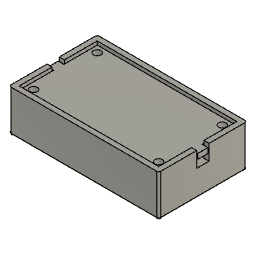
DC-DC Enclosure v1 (Autodesk Fusion 360 design; units mm, degrees)
Autodesk Fusion 360 part; units mm, degrees
sketch "Main geometry layout" plane through (0, 0, 0) normal (0, 0, 1) x (1, 0, 0)
  line L0 (0, 0) -> (61, 0) construction
  line L1 (61, 0) -> (61, 31) construction
  line L2 (61, 31) -> (0, 31) construction
  line L3 (0, 31) -> (0, 0) construction
  circle A0 centre (0, 0) radius 2.75
  circle A1 centre (61, 0) radius 2.75
  circle A2 centre (0, 31) radius 2.75
  circle A3 centre (61, 31) radius 2.75
  line L4 (64.5, 34.5) -> (-3.5, 34.5)
  line L5 (-3.5, 34.5) -> (-3.5, -3.5)
  line L6 (-3.5, -3.5) -> (64.5, -3.5)
  line L7 (64.5, -3.5) -> (64.5, 34.5)
  line L8 (0, 0) -> (9, 0) construction
  line L9 (9, 0) -> (9, 2) construction
  line L10 (9, 2) -> (0, 2) construction
  line L11 (0, 2) -> (0, 0) construction
  circle A4 centre (9, 2) radius 2
  circle A5 centre (29, 31) radius 1.5
  line L12 (-6, -6) -> (67, -6)
  line L13 (67, -6) -> (67, 37)
  line L14 (67, 37) -> (-6, 37)
  line L15 (-6, 37) -> (-6, -6)
  line L16 (-6, 18.5) -> (-3.5, 18.5)
  line L17 (-3.5, 18.5) -> (-3.5, 12.5)
  line L18 (-3.5, 12.5) -> (-6, 12.5)
  line L19 (-6, 12.5) -> (-6, 18.5)
  line L20 (30.5, -13.9919) -> (30.5, 45)
  line L21 (64.5, 18.5) -> (64.5, 12.5)
  line L22 (67, 18.5) -> (64.5, 18.5)
  line L23 (67, 12.5) -> (67, 18.5)
  line L24 (64.5, 12.5) -> (67, 12.5)
  line L25 (-3.5, 34.5) -> (-1.5, 34.5)
  line L26 (-1.5, 34.5) -> (-1.5, 22.5)
  line L27 (-1.5, 22.5) -> (-3.5, 22.5)
  line L28 (-3.5, 22.5) -> (-3.5, 34.5)
  line L29 (72.2627, 15.5) -> (-12, 15.5)
  line L30 (-3.5, -3.5) -> (-1.5, -3.5)
  line L31 (-1.5, -3.5) -> (-1.5, 8.5)
  line L32 (-1.5, 8.5) -> (-3.5, 8.5)
  line L33 (-3.5, 8.5) -> (-3.5, -3.5)
  line L34 (64.5, 34.5) -> (62.5, 34.5)
  line L35 (62.5, 22.5) -> (64.5, 22.5)
  line L36 (64.5, 22.5) -> (64.5, 34.5)
  line L37 (62.5, 34.5) -> (62.5, 22.5)
  line L38 (64.5, 8.5) -> (64.5, -3.5)
  line L39 (64.5, -3.5) -> (62.5, -3.5)
  line L40 (62.5, 8.5) -> (64.5, 8.5)
  line L41 (62.5, -3.5) -> (62.5, 8.5)
  circle A6 centre (9, 2) radius 4.5
  line L42 (18, -1.5) -> (40.5, -1.5)
  line L43 (40.5, -1.5) -> (40.5, 12.5)
  line L44 (40.5, 12.5) -> (18, 12.5)
  line L45 (18, 12.5) -> (18, -1.5)
  line L46 (-1.5, 22.5) -> (-1.5, 8.5)
  line L47 (62.5, 22.5) -> (62.5, 8.5)
  line L48 (13.5, 2) -> (13.5, -3.5)
  line L49 (4.5, 2) -> (4.5, -3.5)
  line L50 (2.75, 0) -> (2.75, -3.5)
  line L51 (2.75, 31) -> (2.75, 34.5)
  line L52 (58.25, 31) -> (58.25, 34.5)
  line L53 (58.25, 0) -> (58.25, -3.5)
  circle A7 centre (0, 0) radius 1.25
  circle A8 centre (61, 0) radius 1.25
  circle A9 centre (0, 31) radius 1.25
  circle A10 centre (61, 31) radius 1.25
  dimension "d1" = 61
  dimension "d2" = 31
  dimension "d6" = 5.5
  dimension "d9" = 61
  dimension "d10" = 31
  dimension "d11" = 3.5
  dimension "d16" = 9
  dimension "d17" = 2
  dimension "d18" = 4
  dimension "d19" = 3
  dimension "d20" = 29
  dimension "d21" = 6
  dimension "d22" = 6
  dimension "d31" = 2
  dimension "d32" = 12
  dimension "d35" = 2.5
  dimension "d40" = 22.5
  dimension "d41" = 14
  dimension "d42" = 18
  dimension "d43" = 2
  dimension "d50" = 2.5
  dimension "d53" = 61
  dimension "d54" = 31
  constraint horizontal L0
  constraint vertical L1
  constraint horizontal L2
  constraint vertical L3
  constraint coincident L0.start L3.end
  constraint horizontal L8
  constraint vertical L9
  constraint horizontal L10
  constraint vertical L11
  constraint coincident L9.end L10.start
  constraint coincident L2 A5.centre
  constraint horizontal L16
  constraint vertical L17
  constraint horizontal L18
  constraint vertical L19
  constraint coincident L15 L16.start
  constraint midpoint L15 L19
  constraint perpendicular L4 L20
  constraint symmetric L16.start L20 L22.start
  constraint symmetric L16.end L20 L21.start
  constraint symmetric L17.end L20 L21.end
  constraint symmetric L18.end L20 L23.start
  constraint horizontal L25
  constraint vertical L26
  constraint horizontal L27
  constraint vertical L28
  constraint perpendicular L21 L29
  constraint symmetric L4.end L29 L5.end
  constraint symmetric L25.end L29 L30.end
  constraint symmetric L26.end L29 L31.end
  constraint symmetric L27.end L29 L32.end
  constraint symmetric L4.end L20 L4.start
  constraint symmetric L20 L25.end L34.end
  constraint symmetric L20 L26.end L35.start
  constraint symmetric L20 L27.end L35.end
  constraint symmetric L20 L5.end L6.end
  constraint symmetric L20 L30.end L39.end
  constraint symmetric L20 L31.end L40.start
  constraint symmetric L20 L32.end L38.start
  constraint horizontal L42
  constraint vertical L43
  constraint horizontal L44
  constraint vertical L45
  constraint coincident A6 L48.start
  constraint coincident L6 L48.end
  constraint tangent A6 L48
  constraint perpendicular L6 L48
  constraint midpoint L10 L49.start
  constraint coincident L6 L49.end
  constraint tangent A6 L49
  constraint perpendicular L6 L49
  constraint coincident A0 L50.start
  constraint coincident L0 L50.start
  constraint coincident L6 L50.end
  constraint tangent A0 L50
  constraint symmetric L29 L50.start L51.start
  constraint symmetric L29 L50.end L51.end
  constraint symmetric L20 L50.start L53.start
  constraint symmetric L20 L50.end L53.end
  constraint symmetric L20 L51.start L52.start
  constraint symmetric L20 L51.end L52.end
  measures "d1" distance of L0.start L0.end
  measures "d2" distance of L0.start L2.end
  measures "d6" diameter of A0
  measures "d16" distance of L0.start L8.end
  measures "d17" distance of L0.start L10.end
  measures "d18" diameter of A4
  measures "d19" diameter of A5
  measures "d20" distance of L2.end A5.centre
  measures "d22" distance of L16.start L18.end
  measures "d31" distance of L4.end L25.end
  measures "d32" distance of L4.end L27.end
  measures "d40" distance of L42.start L42.end
  measures "d41" distance of L42.start L44.end
  measures "d42" distance of L0.start L45
  measures "d43" distance of L6 L42
  measures "d50" diameter of A7
extrude "Extrude1" add sketch "Main geometry layout" against normal blind 2.5 contours A0 L31 | A0 L6 L31 L50 | A0 L6 L20 L29 L31 A6 L42 L44 L45 L46 L48 L49 L50 | A0 L31 | A0 L5 L6 L30 L31 L32 L33 | L5 L6 L12 L15 L18 L20 L30 L33 | L5 L17 L29 L32 L46 | L6 A6 L48 L49 | A2 L4 L20 L26 L29 L46 L51 | L5 L17 L27 L29 L46 | A6 | L5 L15 L17 L18 L19 L29 | A1 L6 L20 L29 L41 L42 L43 L44 L47 L53 | A3 L4 L20 L29 L37 L47 L52 | L5 L15 L16 L17 L19 L29 | A2 L4 L5 L25 L26 L27 L28 | L6 L7 L12 L13 L20 L24 L38 L39 | L20 L42 L43 L44 | L20 L42 L44 L45 | L7 L21 L29 L35 L47 | L7 L21 L29 L40 L47 | L4 L5 L14 L15 L16 L20 L25 L28 | A2 L26 | A2 L26 | A1 L6 L41 L53 | L4 L7 L13 L14 L20 L22 L34 L36 | L7 L13 L21 L23 L24 L29 | L7 L13 L21 L22 L23 L29 | A3 L4 L7 L34 L35 L36 L37 | A1 L6 L7 L38 L39 L40 L41 | A2 L4 L26 L51 | A1 L41 | A3 L4 L37 L52 | A3 L37 | A3 L37 | A1 L41 | A7 | A8 | A9 | A10 makes body 1
extrude "Extrude2" add sketch "Main geometry layout" along normal blind 18 contours L5 L6 L12 L15 L18 L20 L30 L33 | L5 L15 L17 L18 L19 L29 | L5 L15 L16 L17 L19 L29 | L6 L7 L12 L13 L20 L24 L38 L39 | L4 L5 L14 L15 L16 L20 L25 L28 | L4 L7 L13 L14 L20 L22 L34 L36 | L7 L13 L21 L23 L24 L29 | L7 L13 L21 L22 L23 L29 bodies 1
sketch "Cable cutouts" plane through (0, 0, 18) normal (0, 0, 1) x (-1, 0, 0)
  line L0 (3.5, -34.5) -> (-64.5, -34.5)
  line L1 (-64.5, -34.5) -> (-64.5, 3.5)
  line L2 (-64.5, 3.5) -> (3.5, 3.5)
  line L3 (3.5, 3.5) -> (3.5, -34.5)
  line L4 (6, -37) -> (6, 6)
  line L5 (6, 6) -> (-67, 6)
  line L6 (-67, 6) -> (-67, -37)
  line L7 (-67, -37) -> (6, -37)
  line L8 (3.5, -12.5) -> (6, -12.5)
  line L9 (6, -12.5) -> (6, -18.5)
  line L10 (6, -18.5) -> (3.5, -18.5)
  line L11 (3.5, -18.5) -> (3.5, -12.5)
  line L12 (-64.5, -12.5) -> (-67, -12.5)
  line L13 (-67, -12.5) -> (-67, -18.5)
  line L14 (-64.5, -18.5) -> (-64.5, -12.5)
  line L15 (-67, -18.5) -> (-64.5, -18.5)
extrude "Extrude3" cut sketch "Cable cutouts" against normal blind 7.5 contours L3 L4 L8 L9 L10 L11 | L1 L6 L12 L13 L14 L15 bodies 1
fillet "Fillet1" radius 1 8 edges at (30.5, 37, -2.5) (-6, 37, 7.75) (67, 37, 7.75) (67, 15.5, -2.5) (67, -6, 7.75) (30.5, -6, -2.5) (-6, 15.5, -2.5) (-6, -6, 7.75) on bodies 1
extrude "Extrude4" add sketch "Main geometry layout" along normal blind 12 contours A0 L31 | A0 L6 L31 L50 | A0 L31 | A0 L5 L6 L30 L31 L32 L33 | A2 L4 L5 L25 L26 L27 L28 | A2 L26 | A2 L26 | A1 L6 L41 L53 | A3 L4 L7 L34 L35 L36 L37 | A1 L6 L7 L38 L39 L40 L41 | A2 L4 L26 L51 | A1 L41 | A3 L4 L37 L52 | A3 L37 | A3 L37 | A1 L41 | A7 | A8 | A9 | A10 bodies 1
extrude "Extrude5" add sketch "Main geometry layout" along normal blind 5 contours L6 A6 L48 L49 | A6 bodies 1
extrude "Extrude6" cut sketch "Main geometry layout" against normal blind 1.25 contours L20 L42 L43 L44 | L20 L42 L44 L45 bodies 1
fillet "Fillet2" radius 0.5 2 edges at (7.1353, 1.2768, -2.5) (27.6015, 30.4576, -2.5) on bodies 1
extrude "Extrude7" add sketch "Main geometry layout" along normal up to surface (10.5 mm away) contours L5 L17 L29 L32 L46 | L5 L17 L27 L29 L46 | L7 L21 L29 L35 L47 | L7 L21 L29 L40 L47 bodies 1
sketch "Mounting holes" plane through (0, 0, 12) normal (0, 0, 1) x (-1, 0, 0)
  arc A0 (1.5, -28.6951) -> (-2.75, -31) centre (0, -31) ccw
  line L0 (-2.75, -31) -> (-2.75, -34.5)
  line L1 (-2.75, -34.5) -> (3.5, -34.5)
  line L2 (3.5, -34.5) -> (3.5, -22.5)
  line L3 (3.5, -22.5) -> (1.5, -22.5)
  line L4 (1.5, -22.5) -> (1.5, -28.6951)
  circle A1 centre (0, -31) radius 1.25
  circle A2 centre (-61, -31) radius 1.25
  circle A3 centre (-61, 0) radius 1.25
  circle A4 centre (0, 0) radius 1.25
  point P0 (-61, 0)
extrude "Extrude8" cut sketch "Mounting holes" against normal blind 10 contours A1 | A2 | A3 | A4 bodies 1
sketch "Bottom lid" plane through (0, 0, 18) normal (0, 0, 1) x (-1, 0, 0)
  arc A0 (-66, 6) -> (-67, 5) centre (-66, 5) ccw
  line L0 (-67, 5) -> (-67, -12.5)
  line L1 (-67, -12.5) -> (-64.5, -12.5) construction
  line L2 (-64.5, -12.5) -> (-64.5, 3.5)
  line L3 (-64.5, 3.5) -> (3.5, 3.5) construction
  line L4 (3.5, 3.5) -> (3.5, -12.5)
  line L5 (3.5, -12.5) -> (6, -12.5)
  line L6 (6, -12.5) -> (6, 5)
  arc A1 (6, 5) -> (5, 6) centre (5, 5) ccw
  line L7 (5, 6) -> (-66, 6)
  line L8 (-64.5, -34.5) -> (3.5, -34.5) construction
  line L9 (3.5, -34.5) -> (3.5, 3.5) construction
  line L10 (3.5, 3.5) -> (-64.5, 3.5) construction
  line L11 (-64.5, 3.5) -> (-64.5, -34.5) construction
  line L12 (-67, -18.5) -> (-64.5, -18.5) construction
  line L13 (-67, -12.5) -> (-67, -18.5) construction
  line L14 (-64.5, -12.5) -> (-67, -12.5)
  line L15 (6, -18.5) -> (3.5, -18.5) construction
  line L16 (6, -12.5) -> (6, -18.5) construction
  line L17 (3.5, -12.5) -> (6, -12.5) construction
  line L18 (-64.25, -34.25) -> (3.25, -34.25)
  line L19 (3.25, -34.25) -> (3.25, 3.25)
  line L20 (3.25, 3.25) -> (-64.25, 3.25)
  line L21 (-64.25, 3.25) -> (-64.25, -34.25)
  line L22 (6, -18) -> (3.5, -18)
  line L23 (3.5, -13) -> (6, -13)
  line L24 (-67, -18) -> (-64.5, -18)
  line L25 (-67, -13) -> (-64.5, -13)
  line L26 (6, -18) -> (6, -13)
  line L27 (3.5, -18) -> (3.25, -18)
  line L28 (3.5, -13) -> (3.25, -13)
  line L29 (-64.5, -18) -> (-64.25, -18)
  line L30 (-64.5, -13) -> (-64, -13)
  line L31 (-67, -18) -> (-67, -13)
  circle A2 centre (0, 0) radius 1.25 construction
  circle A3 centre (0, 0) radius 1.85
  circle A4 centre (-61, 0) radius 1.85
  circle A5 centre (0, -31) radius 1.85
  circle A6 centre (-61, -31) radius 1.85
  dimension "d57" = -0.25
  dimension "d58" = 0.5
  dimension "d59" = 0.5
  dimension "d60" = -0.5
  dimension "d61" = 0.5
  dimension "d71" = 0.6
  constraint perpendicular L23 L26
  constraint coincident L19 L27.end
  constraint perpendicular L19 L27
  constraint coincident L19 L28.end
  constraint perpendicular L19 L28
  constraint coincident L21 L29.end
  constraint perpendicular L21 L29
  constraint perpendicular L21 L30
  constraint perpendicular L25 L31
extrude "Extrude9" add sketch "Bottom lid" against normal blind 2.5 separate body makes body 2
move_body "Move1" bodies 2 to x (1, 0, 0) y (0, 1, 0) z (0, 0, 1) at (0, 0, -1.5)
equation "d1 = mounting_hole_width"
equation "d2 = mounting_hole_depth"
equation "mounting_hole_width = 61 mm"
equation "mounting_hole_depth = 31 mm"
equation "mounting_hole_diameter = 3 mm"
equation "d6 = mounting_hole_diameter + wall_thickness"
equation "d9 = mounting_hole_width"
equation "d10 = mounting_hole_depth"
equation "d11 = mounting_hole_diameter / 2 + mounting_hole_margin"
equation "mounting_hole_margin = 2 mm"
equation "wall_thickness = 2.5 mm"
equation "pcb_thickness = 2 mm"
equation "tallest_component_height = 12 mm"
equation "d21 = wall_thickness + mounting_hole_diameter / 2 + mounting_hole_margin"
equation "d23 = -wall_thickness"
equation "d25 = tallest_component_height + pcb_thickness + wall_thickness + 1.5 mm"
equation "d27 = -wall_thickness - pcb_thickness - 3 mm"
equation "d33 = tallest_component_height"
equation "d35 = wall_thickness"
equation "d36 = wall_thickness * 2"
equation "display_width = 22.5 mm"
equation "display_height = 14 mm"
equation "d40 = display_width"
equation "d41 = display_height"
equation "d43 = mounting_hole_margin"
equation "d44 = -wall_thickness / 2"
equation "d53 = mounting_hole_width"
equation "d54 = mounting_hole_depth"
equation "d62 = -wall_thickness"
equation "d74 = -mounting_hole_width"
equation "d75 = -mounting_hole_depth"
named bodies: "Main Body", "Bottom lid"
